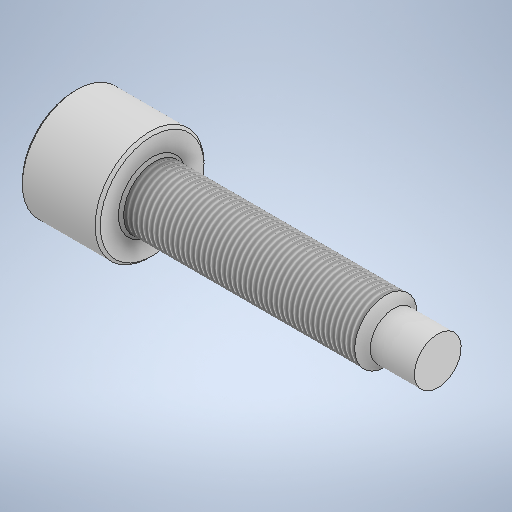
# Autodesk Inventor part: Sroub
Saved by Autodesk Inventor 2025 (Build 290162000, 162)
## iProperties
Created: 2025-04-24
Part Number: Sroub
Material: Všeobecné
Document SubType Name: Modeling
Designer: jakub
Density: 1 g/cm^3
Appearance: Výchozí
Author: jakub
Autodesk Inventor part; units mm, degrees
ref_plane "YZ Plane" through (0, 0, 0) normal (1, 0, 0) x (0, 1, 0)
ref_plane "XZ Plane" through (0, 0, 0) normal (0, 1, 0) x (-1, 0, 0)
ref_plane "XY Plane" through (0, 0, 0) normal (0, 0, 1) x (1, 0, 0)
sketch "Sketch1" plane through (0, 0, 0) normal (0, 0, 1) x (1, 0, 0)
  line L0 (0, 0) -> (0, 10)
  line L1 (0.5, 10.5) -> (14.5, 10.5)
  line L2 (15, 10) -> (15, 6.5)
  line L3 (15, 0) -> (70, 0)
  line L4 (70, 0) -> (70, 4.5)
  line L5 (70, 4.5) -> (61.5, 4.5)
  line L6 (0, 10) -> (0.5, 10.5)
  line L7 (15, 10) -> (14.5, 10.5)
  line L8 (61.5, 4.5) -> (61.5, 4.5)
  line L9 (60, 6) -> (15.5, 6)
  line L10 (15.5, 6) -> (15, 6.5)
  line L11 (60, 6) -> (61.5, 4.5)
  line L12 (0, 0) -> (17, 0)
  point P0 (0, 10.5)
  point P1 (15, 10.5)
  point P2 (61.5, 6)
  point P3 (15, 6)
  point P4 (15, 6)
  constraints: 26 end point, 11 point on line, 4 perpendicular, 2 vertical, 1 horizontal
revolve "Revolution1" add sketch "Sketch1" angle 360 about axis through (0, 0, 0) along (1, 0, 0)
thread "Thread1" size "M12x1" class "6g" standard "ANSI Metric M Profile" full length
body "Solid1"
